Autodesk Fusion 360 part; units mm, degrees
note: some values were not read from the file. Set by a fixed rule: which sketch regions a step uses.
(part 2 of 2)
  spline S32 degree 5 poles (9.6095, -4.902) (9.5996, -4.9074) (9.5799, -4.9184) (9.5504, -4.9349) (9.5113, -4.9571) (9.4627, -4.9851) (9.4143, -5.0134) (9.3662, -5.0419) (9.3184, -5.0706) (9.2709, -5.0997) (9.2236, -5.1289) (9.1767, -5.1585) (9.1301, -5.1883) (9.0838, -5.2184) (9.0377, -5.2487) (8.992, -5.2793) (8.9466, -5.3102) (8.9016, -5.3413) (8.8568, -5.3727) (8.8124, -5.4044) (8.7683, -5.4364) (8.7246, -5.4686) (8.6812, -5.5011) (8.6382, -5.5339) (8.5955, -5.5669) (8.5532, -5.6003) (8.5113, -5.6339) (8.4697, -5.6678) (8.4286, -5.702) (8.3878, -5.7365) (8.3474, -5.7713) (8.3075, -5.8064) (8.268, -5.8419) (8.229, -5.8776) (8.1904, -5.9136) (8.1523, -5.95) (8.1146, -5.9867) (8.0774, -6.0237) (8.0407, -6.0611) (8.0046, -6.0988) (7.9691, -6.1369) (7.9341, -6.1755) (7.8999, -6.2144) (7.8664, -6.2538) (7.8337, -6.2937) (7.8017, -6.3341) (7.7767, -6.3667) (7.7583, -6.3914) (7.7462, -6.408) (7.7402, -6.4163) knots -1 -1 -1 -1 -1 -1 -0.977778 -0.955556 -0.933333 -0.911111 -0.888889 -0.866667 -0.844444 -0.822222 -0.8 -0.777778 -0.755556 -0.733333 -0.711111 -0.688889 -0.666667 -0.644444 -0.622222 -0.6 -0.577778 -0.555556 -0.533333 -0.511111 -0.488889 -0.466667 -0.444444 -0.422222 -0.4 -0.377778 -0.355556 -0.333333 -0.311111 -0.288889 -0.266667 -0.244444 -0.222222 -0.2 -0.177778 -0.155556 -0.133333 -0.111111 -0.088889 -0.066667 -0.044444 -0.022222 0 0 0 0 0 0
  arc A33 (7.7402, -6.4163) -> (6.5319, -5.8168) centre (0, -20.5) ccw
  spline S33 degree 5 poles (6.5319, -5.8168) (6.5348, -5.807) (6.5407, -5.7873) (6.5493, -5.7577) (6.5602, -5.7181) (6.5729, -5.6682) (6.5849, -5.618) (6.596, -5.5675) (6.6063, -5.5167) (6.6159, -5.4656) (6.6247, -5.4142) (6.6329, -5.3626) (6.6405, -5.3108) (6.6475, -5.2588) (6.6539, -5.2066) (6.6598, -5.1543) (6.6652, -5.1017) (6.67, -5.049) (6.6743, -4.9962) (6.6781, -4.9431) (6.6814, -4.8899) (6.6842, -4.8366) (6.6865, -4.7831) (6.6884, -4.7295) (6.6898, -4.6758) (6.6908, -4.6219) (6.6913, -4.568) (6.6914, -4.5139) (6.691, -4.4597) (6.6902, -4.4053) (6.689, -4.3509) (6.6873, -4.2964) (6.6853, -4.2418) (6.6828, -4.187) (6.6799, -4.1322) (6.6766, -4.0773) (6.6729, -4.0223) (6.6689, -3.9672) (6.6644, -3.9121) (6.6595, -3.8568) (6.6543, -3.8015) (6.6486, -3.7461) (6.6426, -3.6906) (6.6362, -3.6351) (6.6295, -3.5795) (6.6223, -3.5238) (6.6163, -3.4792) (6.6117, -3.4458) (6.6085, -3.4234) (6.6068, -3.4123) knots 0 0 0 0 0 0 0.022222 0.044444 0.066667 0.088889 0.111111 0.133333 0.155556 0.177778 0.2 0.222222 0.244444 0.266667 0.288889 0.311111 0.333333 0.355556 0.377778 0.4 0.422222 0.444444 0.466667 0.488889 0.511111 0.533333 0.555556 0.577778 0.6 0.622222 0.644444 0.666667 0.688889 0.711111 0.733333 0.755556 0.777778 0.8 0.822222 0.844444 0.866667 0.888889 0.911111 0.933333 0.955556 0.977778 1 1 1 1 1 1
  arc A34 (6.6068, -3.4123) -> (6.1565, -3.2449) centre (0, -20.5) ccw
  spline S34 degree 5 poles (6.1565, -3.2449) (6.148, -3.2523) (6.131, -3.2671) (6.1056, -3.2894) (6.0719, -3.3193) (6.0301, -3.3568) (5.9887, -3.3944) (5.9476, -3.4323) (5.9068, -3.4704) (5.8664, -3.5087) (5.8263, -3.5471) (5.7865, -3.5858) (5.7471, -3.6247) (5.708, -3.6637) (5.6693, -3.703) (5.631, -3.7424) (5.593, -3.782) (5.5554, -3.8219) (5.5181, -3.8619) (5.4813, -3.9021) (5.4448, -3.9425) (5.4087, -3.9831) (5.3731, -4.0239) (5.3378, -4.0649) (5.3029, -4.1062) (5.2685, -4.1476) (5.2344, -4.1892) (5.2009, -4.231) (5.1677, -4.273) (5.135, -4.3152) (5.1028, -4.3577) (5.071, -4.4003) (5.0397, -4.4431) (5.009, -4.4862) (4.9787, -4.5295) (4.949, -4.573) (4.9198, -4.6167) (4.8911, -4.6607) (4.863, -4.7049) (4.8355, -4.7493) (4.8087, -4.794) (4.7825, -4.8389) (4.7571, -4.8841) (4.7326, -4.9296) (4.7088, -4.9754) (4.6859, -5.0216) (4.6683, -5.0587) (4.6554, -5.0867) (4.6471, -5.1054) (4.6429, -5.1148) knots -1 -1 -1 -1 -1 -1 -0.977778 -0.955556 -0.933333 -0.911111 -0.888889 -0.866667 -0.844444 -0.822222 -0.8 -0.777778 -0.755556 -0.733333 -0.711111 -0.688889 -0.666667 -0.644444 -0.622222 -0.6 -0.577778 -0.555556 -0.533333 -0.511111 -0.488889 -0.466667 -0.444444 -0.422222 -0.4 -0.377778 -0.355556 -0.333333 -0.311111 -0.288889 -0.266667 -0.244444 -0.222222 -0.2 -0.177778 -0.155556 -0.133333 -0.111111 -0.088889 -0.066667 -0.044444 -0.022222 0 0 0 0 0 0
  arc A35 (4.6429, -5.1148) -> (3.3363, -4.7796) centre (0, -20.5) ccw
  spline S35 degree 5 poles (3.3363, -4.7796) (3.3372, -4.7694) (3.3389, -4.749) (3.3411, -4.7182) (3.3435, -4.6772) (3.3456, -4.6257) (3.3469, -4.5742) (3.3472, -4.5224) (3.3467, -4.4706) (3.3455, -4.4186) (3.3434, -4.3665) (3.3407, -4.3144) (3.3373, -4.2621) (3.3334, -4.2098) (3.3288, -4.1574) (3.3237, -4.105) (3.318, -4.0525) (3.3118, -3.9999) (3.305, -3.9473) (3.2977, -3.8946) (3.2899, -3.8419) (3.2815, -3.7892) (3.2727, -3.7364) (3.2634, -3.6836) (3.2536, -3.6307) (3.2433, -3.5778) (3.2326, -3.5249) (3.2214, -3.472) (3.2098, -3.4191) (3.1977, -3.3661) (3.1852, -3.3131) (3.1723, -3.2601) (3.1589, -3.2071) (3.1451, -3.1541) (3.1309, -3.1011) (3.1163, -3.048) (3.1012, -2.995) (3.0858, -2.942) (3.0699, -2.8889) (3.0537, -2.8359) (3.0371, -2.7829) (3.02, -2.7299) (3.0026, -2.6769) (2.9848, -2.6239) (2.9666, -2.5709) (2.9481, -2.5179) (2.9329, -2.4756) (2.9214, -2.4438) (2.9136, -2.4226) (2.9097, -2.412) knots 0 0 0 0 0 0 0.022222 0.044444 0.066667 0.088889 0.111111 0.133333 0.155556 0.177778 0.2 0.222222 0.244444 0.266667 0.288889 0.311111 0.333333 0.355556 0.377778 0.4 0.422222 0.444444 0.466667 0.488889 0.511111 0.533333 0.555556 0.577778 0.6 0.622222 0.644444 0.666667 0.688889 0.711111 0.733333 0.755556 0.777778 0.8 0.822222 0.844444 0.866667 0.888889 0.911111 0.933333 0.955556 0.977778 1 1 1 1 1 1
  arc A36 (2.9097, -2.412) -> (2.4344, -2.342) centre (0, -20.5) ccw
  spline S36 degree 5 poles (2.4344, -2.342) (2.4276, -2.351) (2.4141, -2.369) (2.3939, -2.3961) (2.3671, -2.4323) (2.3341, -2.4776) (2.3014, -2.5231) (2.2691, -2.5687) (2.2371, -2.6144) (2.2055, -2.6603) (2.1742, -2.7063) (2.1434, -2.7523) (2.1129, -2.7985) (2.0828, -2.8449) (2.0531, -2.8913) (2.0238, -2.9378) (1.9949, -2.9845) (1.9664, -3.0313) (1.9383, -3.0782) (1.9106, -3.1252) (1.8833, -3.1723) (1.8565, -3.2195) (1.8301, -3.2669) (1.8041, -3.3143) (1.7786, -3.3619) (1.7535, -3.4095) (1.7288, -3.4573) (1.7047, -3.5052) (1.681, -3.5532) (1.6578, -3.6013) (1.6351, -3.6495) (1.6129, -3.6978) (1.5912, -3.7462) (1.5701, -3.7947) (1.5495, -3.8434) (1.5294, -3.8921) (1.51, -3.9409) (1.4911, -3.9899) (1.4727, -4.039) (1.4551, -4.0881) (1.4381, -4.1374) (1.4219, -4.1868) (1.4065, -4.2363) (1.3919, -4.2859) (1.3782, -4.3357) (1.3654, -4.3855) (1.3559, -4.4255) (1.3491, -4.4556) (1.3448, -4.4756) (1.3427, -4.4857) knots -1 -1 -1 -1 -1 -1 -0.977778 -0.955556 -0.933333 -0.911111 -0.888889 -0.866667 -0.844444 -0.822222 -0.8 -0.777778 -0.755556 -0.733333 -0.711111 -0.688889 -0.666667 -0.644444 -0.622222 -0.6 -0.577778 -0.555556 -0.533333 -0.511111 -0.488889 -0.466667 -0.444444 -0.422222 -0.4 -0.377778 -0.355556 -0.333333 -0.311111 -0.288889 -0.266667 -0.244444 -0.222222 -0.2 -0.177778 -0.155556 -0.133333 -0.111111 -0.088889 -0.066667 -0.044444 -0.022222 0 0 0 0 0 0
  arc A37 (1.3427, -4.4857) -> (-0.005, -4.4295) centre (0, -20.5) ccw
  spline S37 degree 5 poles (-0.005, -4.4295) (-0.0063, -4.4193) (-0.0089, -4.399) (-0.0132, -4.3685) (-0.0193, -4.3278) (-0.0279, -4.277) (-0.0375, -4.2263) (-0.0478, -4.1757) (-0.0591, -4.125) (-0.0711, -4.0745) (-0.084, -4.024) (-0.0975, -3.9735) (-0.1116, -3.9231) (-0.1264, -3.8727) (-0.1417, -3.8224) (-0.1577, -3.7722) (-0.1741, -3.722) (-0.1911, -3.6719) (-0.2087, -3.6218) (-0.2268, -3.5719) (-0.2454, -3.5219) (-0.2646, -3.4721) (-0.2842, -3.4223) (-0.3043, -3.3725) (-0.3248, -3.3229) (-0.3459, -3.2733) (-0.3674, -3.2238) (-0.3893, -3.1743) (-0.4117, -3.125) (-0.4345, -3.0757) (-0.4577, -3.0264) (-0.4814, -2.9773) (-0.5055, -2.9282) (-0.53, -2.8792) (-0.555, -2.8303) (-0.5803, -2.7815) (-0.606, -2.7328) (-0.6322, -2.6841) (-0.6587, -2.6355) (-0.6856, -2.587) (-0.7129, -2.5386) (-0.7406, -2.4903) (-0.7686, -2.4421) (-0.7971, -2.3939) (-0.8259, -2.3459) (-0.855, -2.2979) (-0.8787, -2.2597) (-0.8965, -2.231) (-0.9085, -2.2119) (-0.9146, -2.2023) knots 0 0 0 0 0 0 0.022222 0.044444 0.066667 0.088889 0.111111 0.133333 0.155556 0.177778 0.2 0.222222 0.244444 0.266667 0.288889 0.311111 0.333333 0.355556 0.377778 0.4 0.422222 0.444444 0.466667 0.488889 0.511111 0.533333 0.555556 0.577778 0.6 0.622222 0.644444 0.666667 0.688889 0.711111 0.733333 0.755556 0.777778 0.8 0.822222 0.844444 0.866667 0.888889 0.911111 0.933333 0.955556 0.977778 1 1 1 1 1 1
  arc A38 (-0.9146, -2.2023) -> (-1.394, -2.2326) centre (0, -20.5) ccw
  spline S38 degree 5 poles (-1.394, -2.2326) (-1.3988, -2.2428) (-1.4083, -2.2633) (-1.4224, -2.294) (-1.4411, -2.3349) (-1.464, -2.3862) (-1.4865, -2.4375) (-1.5087, -2.4888) (-1.5304, -2.5402) (-1.5518, -2.5916) (-1.5728, -2.643) (-1.5934, -2.6945) (-1.6136, -2.7461) (-1.6334, -2.7976) (-1.6528, -2.8492) (-1.6718, -2.9008) (-1.6904, -2.9525) (-1.7085, -3.0042) (-1.7263, -3.0559) (-1.7436, -3.1076) (-1.7605, -3.1594) (-1.7769, -3.2112) (-1.7929, -3.263) (-1.8084, -3.3148) (-1.8235, -3.3666) (-1.8381, -3.4184) (-1.8523, -3.4703) (-1.866, -3.5221) (-1.8792, -3.574) (-1.8919, -3.6259) (-1.9041, -3.6778) (-1.9158, -3.7296) (-1.9269, -3.7815) (-1.9375, -3.8334) (-1.9475, -3.8852) (-1.957, -3.937) (-1.9659, -3.9889) (-1.9742, -4.0407) (-1.9819, -4.0925) (-1.9889, -4.1442) (-1.9953, -4.196) (-2.0009, -4.2476) (-2.0057, -4.2993) (-2.0096, -4.3508) (-2.0127, -4.4023) (-2.0148, -4.4538) (-2.0158, -4.4949) (-2.0162, -4.5257) (-2.0163, -4.5462) (-2.0162, -4.5565) knots -1 -1 -1 -1 -1 -1 -0.977778 -0.955556 -0.933333 -0.911111 -0.888889 -0.866667 -0.844444 -0.822222 -0.8 -0.777778 -0.755556 -0.733333 -0.711111 -0.688889 -0.666667 -0.644444 -0.622222 -0.6 -0.577778 -0.555556 -0.533333 -0.511111 -0.488889 -0.466667 -0.444444 -0.422222 -0.4 -0.377778 -0.355556 -0.333333 -0.311111 -0.288889 -0.266667 -0.244444 -0.222222 -0.2 -0.177778 -0.155556 -0.133333 -0.111111 -0.088889 -0.066667 -0.044444 -0.022222 0 0 0 0 0 0
  arc A39 (-2.0162, -4.5565) -> (-3.3462, -4.7817) centre (0, -20.5) ccw
  spline S39 degree 5 poles (-3.3462, -4.7817) (-3.3495, -4.772) (-3.3563, -4.7527) (-3.3668, -4.7237) (-3.3813, -4.6852) (-3.4003, -4.6374) (-3.4201, -4.5897) (-3.4408, -4.5423) (-3.4623, -4.4952) (-3.4847, -4.4482) (-3.5077, -4.4014) (-3.5314, -4.3549) (-3.5557, -4.3085) (-3.5806, -4.2624) (-3.6061, -4.2163) (-3.6321, -4.1705) (-3.6587, -4.1249) (-3.6857, -4.0794) (-3.7133, -4.0341) (-3.7414, -3.9889) (-3.77, -3.944) (-3.7991, -3.8992) (-3.8286, -3.8545) (-3.8586, -3.8101) (-3.8891, -3.7658) (-3.9199, -3.7216) (-3.9513, -3.6777) (-3.983, -3.6339) (-4.0151, -3.5902) (-4.0477, -3.5468) (-4.0807, -3.5034) (-4.1141, -3.4603) (-4.1479, -3.4173) (-4.182, -3.3745) (-4.2166, -3.3318) (-4.2515, -3.2893) (-4.2868, -3.247) (-4.3225, -3.2048) (-4.3585, -3.1628) (-4.3949, -3.121) (-4.4317, -3.0793) (-4.4688, -3.0378) (-4.5063, -2.9965) (-4.5441, -2.9553) (-4.5823, -2.9143) (-4.6208, -2.8735) (-4.6518, -2.8409) (-4.6753, -2.8166) (-4.691, -2.8004) (-4.6989, -2.7923) knots 0 0 0 0 0 0 0.022222 0.044444 0.066667 0.088889 0.111111 0.133333 0.155556 0.177778 0.2 0.222222 0.244444 0.266667 0.288889 0.311111 0.333333 0.355556 0.377778 0.4 0.422222 0.444444 0.466667 0.488889 0.511111 0.533333 0.555556 0.577778 0.6 0.622222 0.644444 0.666667 0.688889 0.711111 0.733333 0.755556 0.777778 0.8 0.822222 0.844444 0.866667 0.888889 0.911111 0.933333 0.955556 0.977778 1 1 1 1 1 1
  arc A40 (-4.6989, -2.7923) -> (-5.1616, -2.9216) centre (0, -20.5) ccw
  spline S40 degree 5 poles (-5.1616, -2.9216) (-5.1641, -2.9326) (-5.1692, -2.9546) (-5.1766, -2.9876) (-5.1863, -3.0315) (-5.1981, -3.0864) (-5.2094, -3.1412) (-5.2204, -3.1961) (-5.231, -3.2508) (-5.2413, -3.3056) (-5.2511, -3.3603) (-5.2605, -3.4149) (-5.2696, -3.4695) (-5.2782, -3.5241) (-5.2865, -3.5786) (-5.2943, -3.633) (-5.3018, -3.6874) (-5.3088, -3.7417) (-5.3154, -3.796) (-5.3216, -3.8502) (-5.3273, -3.9043) (-5.3326, -3.9584) (-5.3375, -4.0124) (-5.3419, -4.0663) (-5.3459, -4.1201) (-5.3494, -4.1739) (-5.3525, -4.2275) (-5.3551, -4.2811) (-5.3572, -4.3346) (-5.3589, -4.388) (-5.36, -4.4412) (-5.3606, -4.4944) (-5.3607, -4.5475) (-5.3603, -4.6004) (-5.3593, -4.6532) (-5.3578, -4.7059) (-5.3558, -4.7584) (-5.3531, -4.8108) (-5.3499, -4.8631) (-5.346, -4.9152) (-5.3415, -4.9671) (-5.3362, -5.0188) (-5.3302, -5.0703) (-5.3233, -5.1216) (-5.3156, -5.1726) (-5.307, -5.2234) (-5.2994, -5.2638) (-5.2934, -5.294) (-5.2892, -5.314) (-5.287, -5.3241) knots -1 -1 -1 -1 -1 -1 -0.977778 -0.955556 -0.933333 -0.911111 -0.888889 -0.866667 -0.844444 -0.822222 -0.8 -0.777778 -0.755556 -0.733333 -0.711111 -0.688889 -0.666667 -0.644444 -0.622222 -0.6 -0.577778 -0.555556 -0.533333 -0.511111 -0.488889 -0.466667 -0.444444 -0.422222 -0.4 -0.377778 -0.355556 -0.333333 -0.311111 -0.288889 -0.266667 -0.244444 -0.222222 -0.2 -0.177778 -0.155556 -0.133333 -0.111111 -0.088889 -0.066667 -0.044444 -0.022222 0 0 0 0 0 0
  arc A41 (-5.287, -5.3241) -> (-6.5411, -5.8209) centre (0, -20.5) ccw
  spline S41 degree 5 poles (-6.5411, -5.8209) (-6.5464, -5.8121) (-6.557, -5.7946) (-6.5733, -5.7685) (-6.5955, -5.7338) (-6.624, -5.691) (-6.6533, -5.6485) (-6.6834, -5.6064) (-6.7143, -5.5648) (-6.7459, -5.5235) (-6.7781, -5.4825) (-6.811, -5.4419) (-6.8444, -5.4016) (-6.8784, -5.3616) (-6.9129, -5.3219) (-6.9478, -5.2825) (-6.9833, -5.2434) (-7.0192, -5.2045) (-7.0556, -5.1659) (-7.0925, -5.1276) (-7.1298, -5.0896) (-7.1676, -5.0518) (-7.2057, -5.0143) (-7.2443, -4.977) (-7.2833, -4.94) (-7.3227, -4.9033) (-7.3625, -4.8668) (-7.4026, -4.8306) (-7.4431, -4.7946) (-7.484, -4.7588) (-7.5253, -4.7233) (-7.5669, -4.688) (-7.6089, -4.653) (-7.6512, -4.6182) (-7.6939, -4.5837) (-7.7369, -4.5494) (-7.7802, -4.5153) (-7.8239, -4.4815) (-7.8679, -4.4479) (-7.9122, -4.4145) (-7.9568, -4.3814) (-8.0018, -4.3485) (-8.047, -4.3159) (-8.0926, -4.2835) (-8.1384, -4.2513) (-8.1846, -4.2194) (-8.2217, -4.194) (-8.2497, -4.1751) (-8.2684, -4.1625) (-8.2778, -4.1562) knots 0 0 0 0 0 0 0.022222 0.044444 0.066667 0.088889 0.111111 0.133333 0.155556 0.177778 0.2 0.222222 0.244444 0.266667 0.288889 0.311111 0.333333 0.355556 0.377778 0.4 0.422222 0.444444 0.466667 0.488889 0.511111 0.533333 0.555556 0.577778 0.6 0.622222 0.644444 0.666667 0.688889 0.711111 0.733333 0.755556 0.777778 0.8 0.822222 0.844444 0.866667 0.888889 0.911111 0.933333 0.955556 0.977778 1 1 1 1 1 1
  arc A42 (-8.2778, -4.1562) -> (-8.7035, -4.3789) centre (0, -20.5) ccw
  spline S42 degree 5 poles (-8.7035, -4.3789) (-8.7037, -4.3902) (-8.7041, -4.4127) (-8.7045, -4.4465) (-8.7049, -4.4915) (-8.705, -4.5477) (-8.7047, -4.6037) (-8.704, -4.6596) (-8.703, -4.7154) (-8.7016, -4.771) (-8.6999, -4.8266) (-8.6978, -4.882) (-8.6953, -4.9373) (-8.6924, -4.9924) (-8.6891, -5.0475) (-8.6855, -5.1023) (-8.6814, -5.1571) (-8.677, -5.2117) (-8.6722, -5.2661) (-8.667, -5.3204) (-8.6613, -5.3746) (-8.6553, -5.4286) (-8.6488, -5.4824) (-8.642, -5.5361) (-8.6347, -5.5895) (-8.6269, -5.6429) (-8.6188, -5.696) (-8.6102, -5.7489) (-8.6011, -5.8017) (-8.5917, -5.8542) (-8.5817, -5.9066) (-8.5713, -5.9587) (-8.5603, -6.0106) (-8.5489, -6.0623) (-8.537, -6.1137) (-8.5245, -6.1649) (-8.5116, -6.2159) (-8.4981, -6.2666) (-8.4841, -6.3171) (-8.4695, -6.3672) (-8.4542, -6.4171) (-8.4383, -6.4666) (-8.4217, -6.5157) (-8.4043, -6.5644) (-8.3862, -6.6127) (-8.3672, -6.6606) (-8.3514, -6.6985) (-8.3392, -6.7268) (-8.3309, -6.7456) (-8.3267, -6.7549) knots -1 -1 -1 -1 -1 -1 -0.977778 -0.955556 -0.933333 -0.911111 -0.888889 -0.866667 -0.844444 -0.822222 -0.8 -0.777778 -0.755556 -0.733333 -0.711111 -0.688889 -0.666667 -0.644444 -0.622222 -0.6 -0.577778 -0.555556 -0.533333 -0.511111 -0.488889 -0.466667 -0.444444 -0.422222 -0.4 -0.377778 -0.355556 -0.333333 -0.311111 -0.288889 -0.266667 -0.244444 -0.222222 -0.2 -0.177778 -0.155556 -0.133333 -0.111111 -0.088889 -0.066667 -0.044444 -0.022222 0 0 0 0 0 0
  arc A43 (-8.3267, -6.7549) -> (-9.4501, -7.5016) centre (0, -20.5) ccw
  spline S43 degree 5 poles (-9.4501, -7.5016) (-9.4571, -7.4942) (-9.4712, -7.4792) (-9.4925, -7.457) (-9.5214, -7.4278) (-9.5582, -7.3918) (-9.5957, -7.3563) (-9.6339, -7.3214) (-9.6728, -7.2871) (-9.7122, -7.2533) (-9.7523, -7.2199) (-9.7929, -7.1871) (-9.834, -7.1546) (-9.8755, -7.1225) (-9.9175, -7.0909) (-9.9599, -7.0596) (-10.0027, -7.0287) (-10.0459, -6.9981) (-10.0896, -6.968) (-10.1336, -6.9382) (-10.178, -6.9087) (-10.2228, -6.8796) (-10.2679, -6.8509) (-10.3134, -6.8224) (-10.3593, -6.7944) (-10.4054, -6.7666) (-10.4519, -6.7392) (-10.4987, -6.7121) (-10.5458, -6.6853) (-10.5933, -6.6588) (-10.641, -6.6326) (-10.6891, -6.6068) (-10.7374, -6.5813) (-10.786, -6.5561) (-10.835, -6.5311) (-10.8842, -6.5065) (-10.9336, -6.4822) (-10.9834, -6.4582) (-11.0334, -6.4345) (-11.0837, -6.4111) (-11.1342, -6.388) (-11.185, -6.3652) (-11.236, -6.3426) (-11.2873, -6.3204) (-11.3389, -6.2985) (-11.3906, -6.2768) (-11.4323, -6.2597) (-11.4636, -6.247) (-11.4845, -6.2386) (-11.495, -6.2344) knots 0 0 0 0 0 0 0.022222 0.044444 0.066667 0.088889 0.111111 0.133333 0.155556 0.177778 0.2 0.222222 0.244444 0.266667 0.288889 0.311111 0.333333 0.355556 0.377778 0.4 0.422222 0.444444 0.466667 0.488889 0.511111 0.533333 0.555556 0.577778 0.6 0.622222 0.644444 0.666667 0.688889 0.711111 0.733333 0.755556 0.777778 0.8 0.822222 0.844444 0.866667 0.888889 0.911111 0.933333 0.955556 0.977778 1 1 1 1 1 1
  arc A44 (-11.495, -6.2344) -> (-11.8651, -6.5408) centre (0, -20.5) ccw
  spline S44 degree 5 poles (-11.8651, -6.5408) (-11.863, -6.5518) (-11.8586, -6.574) (-11.852, -6.6071) (-11.843, -6.6512) (-11.8314, -6.7061) (-11.8195, -6.7609) (-11.8072, -6.8154) (-11.7947, -6.8697) (-11.7817, -6.9239) (-11.7685, -6.9779) (-11.7549, -7.0316) (-11.7409, -7.0852) (-11.7266, -7.1386) (-11.712, -7.1917) (-11.697, -7.2446) (-11.6817, -7.2973) (-11.666, -7.3498) (-11.65, -7.4021) (-11.6336, -7.4541) (-11.6168, -7.5059) (-11.5997, -7.5575) (-11.5822, -7.6088) (-11.5643, -7.6598) (-11.546, -7.7106) (-11.5274, -7.7612) (-11.5084, -7.8114) (-11.489, -7.8614) (-11.4691, -7.9111) (-11.4489, -7.9606) (-11.4283, -8.0097) (-11.4073, -8.0585) (-11.3858, -8.107) (-11.3639, -8.1552) (-11.3415, -8.2031) (-11.3187, -8.2506) (-11.2954, -8.2977) (-11.2717, -8.3445) (-11.2475, -8.3909) (-11.2228, -8.437) (-11.1975, -8.4826) (-11.1717, -8.5277) (-11.1452, -8.5722) (-11.1181, -8.6163) (-11.0903, -8.6597) (-11.0618, -8.7026) (-11.0384, -8.7365) (-11.0206, -8.7616) (-11.0086, -8.7782) (-11.0025, -8.7865) knots -1 -1 -1 -1 -1 -1 -0.977778 -0.955556 -0.933333 -0.911111 -0.888889 -0.866667 -0.844444 -0.822222 -0.8 -0.777778 -0.755556 -0.733333 -0.711111 -0.688889 -0.666667 -0.644444 -0.622222 -0.6 -0.577778 -0.555556 -0.533333 -0.511111 -0.488889 -0.466667 -0.444444 -0.422222 -0.4 -0.377778 -0.355556 -0.333333 -0.311111 -0.288889 -0.266667 -0.244444 -0.222222 -0.2 -0.177778 -0.155556 -0.133333 -0.111111 -0.088889 -0.066667 -0.044444 -0.022222 0 0 0 0 0 0
  arc A45 (-11.0025, -8.7865) -> (-11.9461, -9.7505) centre (0, -20.5) ccw
  spline S45 degree 5 poles (-11.9461, -9.7505) (-11.9545, -9.7446) (-11.9714, -9.7329) (-11.9969, -9.7157) (-12.0312, -9.6931) (-12.0747, -9.6655) (-12.1188, -9.6386) (-12.1634, -9.6124) (-12.2085, -9.5869) (-12.2542, -9.562) (-12.3003, -9.5378) (-12.3468, -9.514) (-12.3937, -9.4908) (-12.441, -9.4681) (-12.4887, -9.4459) (-12.5367, -9.4241) (-12.585, -9.4027) (-12.6336, -9.3819) (-12.6826, -9.3614) (-12.7318, -9.3414) (-12.7814, -9.3218) (-12.8312, -9.3027) (-12.8814, -9.2839) (-12.9318, -9.2656) (-12.9824, -9.2477) (-13.0334, -9.2301) (-13.0845, -9.2129) (-13.136, -9.1962) (-13.1876, -9.1798) (-13.2395, -9.1637) (-13.2917, -9.1481) (-13.344, -9.1328) (-13.3966, -9.1179) (-13.4495, -9.1033) (-13.5025, -9.0891) (-13.5557, -9.0753) (-13.6092, -9.0618) (-13.6628, -9.0486) (-13.7167, -9.0358) (-13.7707, -9.0234) (-13.8249, -9.0113) (-13.8794, -8.9995) (-13.934, -8.9881) (-13.9888, -8.977) (-14.0437, -8.9663) (-14.0989, -8.9559) (-14.1432, -8.9478) (-14.1764, -8.9419) (-14.1987, -8.938) (-14.2098, -8.9361) knots 0 0 0 0 0 0 0.022222 0.044444 0.066667 0.088889 0.111111 0.133333 0.155556 0.177778 0.2 0.222222 0.244444 0.266667 0.288889 0.311111 0.333333 0.355556 0.377778 0.4 0.422222 0.444444 0.466667 0.488889 0.511111 0.533333 0.555556 0.577778 0.6 0.622222 0.644444 0.666667 0.688889 0.711111 0.733333 0.755556 0.777778 0.8 0.822222 0.844444 0.866667 0.888889 0.911111 0.933333 0.955556 0.977778 1 1 1 1 1 1
  arc A46 (-14.2098, -8.9361) -> (-14.5081, -9.3127) centre (0, -20.5) ccw
  spline S46 degree 5 poles (-14.5081, -9.3127) (-14.5037, -9.3231) (-14.4949, -9.3438) (-14.4815, -9.3749) (-14.4635, -9.4161) (-14.4408, -9.4674) (-14.4177, -9.5185) (-14.3944, -9.5693) (-14.3708, -9.6199) (-14.3469, -9.6701) (-14.3227, -9.7202) (-14.2982, -9.7699) (-14.2735, -9.8194) (-14.2484, -9.8686) (-14.223, -9.9176) (-14.1974, -9.9662) (-14.1714, -10.0146) (-14.1452, -10.0627) (-14.1186, -10.1105) (-14.0917, -10.158) (-14.0646, -10.2051) (-14.0371, -10.252) (-14.0093, -10.2985) (-13.9812, -10.3448) (-13.9528, -10.3907) (-13.924, -10.4362) (-13.895, -10.4814) (-13.8656, -10.5263) (-13.8359, -10.5708) (-13.8058, -10.615) (-13.7754, -10.6587) (-13.7447, -10.7021) (-13.7136, -10.7451) (-13.6821, -10.7877) (-13.6503, -10.8298) (-13.6181, -10.8715) (-13.5856, -10.9128) (-13.5526, -10.9537) (-13.5193, -10.994) (-13.4856, -11.0339) (-13.4514, -11.0733) (-13.4167, -11.112) (-13.3816, -11.1501) (-13.3459, -11.1875) (-13.3096, -11.2243) (-13.2728, -11.2603) (-13.243, -11.2886) (-13.2203, -11.3094) (-13.2051, -11.3232) (-13.1975, -11.3301) knots -1 -1 -1 -1 -1 -1 -0.977778 -0.955556 -0.933333 -0.911111 -0.888889 -0.866667 -0.844444 -0.822222 -0.8 -0.777778 -0.755556 -0.733333 -0.711111 -0.688889 -0.666667 -0.644444 -0.622222 -0.6 -0.577778 -0.555556 -0.533333 -0.511111 -0.488889 -0.466667 -0.444444 -0.422222 -0.4 -0.377778 -0.355556 -0.333333 -0.311111 -0.288889 -0.266667 -0.244444 -0.222222 -0.2 -0.177778 -0.155556 -0.133333 -0.111111 -0.088889 -0.066667 -0.044444 -0.022222 0 0 0 0 0 0
  arc A47 (-13.1975, -11.3301) -> (-13.92, -12.4691) centre (0, -20.5) ccw
  spline S47 degree 5 poles (-13.92, -12.4691) (-13.9294, -12.4651) (-13.9484, -12.4572) (-13.9769, -12.4456) (-14.0152, -12.4306) (-14.0635, -12.4127) (-14.1121, -12.3956) (-14.1612, -12.3793) (-14.2107, -12.3637) (-14.2605, -12.3488) (-14.3107, -12.3347) (-14.3611, -12.3212) (-14.4118, -12.3082) (-14.4628, -12.2958) (-14.5141, -12.284) (-14.5655, -12.2726) (-14.6172, -12.2618) (-14.6691, -12.2515) (-14.7213, -12.2417) (-14.7736, -12.2323) (-14.8262, -12.2235) (-14.8789, -12.2151) (-14.9318, -12.2072) (-14.9849, -12.1998) (-15.0382, -12.1928) (-15.0917, -12.1862) (-15.1453, -12.18) (-15.1991, -12.1743) (-15.2531, -12.169) (-15.3072, -12.1641) (-15.3614, -12.1596) (-15.4158, -12.1556) (-15.4704, -12.1519) (-15.5251, -12.1487) (-15.5799, -12.1458) (-15.6348, -12.1433) (-15.6899, -12.1412) (-15.7451, -12.1395) (-15.8004, -12.1382) (-15.8559, -12.1373) (-15.9115, -12.1367) (-15.9671, -12.1365) (-16.0229, -12.1367) (-16.0788, -12.1372) (-16.1348, -12.1382) (-16.191, -12.1394) (-16.2359, -12.1408) (-16.2697, -12.1419) (-16.2922, -12.1428) (-16.3035, -12.1432) knots 0 0 0 0 0 0 0.022222 0.044444 0.066667 0.088889 0.111111 0.133333 0.155556 0.177778 0.2 0.222222 0.244444 0.266667 0.288889 0.311111 0.333333 0.355556 0.377778 0.4 0.422222 0.444444 0.466667 0.488889 0.511111 0.533333 0.555556 0.577778 0.6 0.622222 0.644444 0.666667 0.688889 0.711111 0.733333 0.755556 0.777778 0.8 0.822222 0.844444 0.866667 0.888889 0.911111 0.933333 0.955556 0.977778 1 1 1 1 1 1
  arc A48 (-16.3035, -12.1432) -> (-16.5171, -12.5736) centre (0, -20.5) ccw
  spline S48 degree 5 poles (-16.5171, -12.5736) (-16.5106, -12.5828) (-16.4976, -12.6013) (-16.4781, -12.6289) (-16.4519, -12.6655) (-16.419, -12.7109) (-16.3859, -12.7561) (-16.3525, -12.8009) (-16.3189, -12.8455) (-16.285, -12.8897) (-16.251, -12.9336) (-16.2167, -12.9772) (-16.1822, -13.0204) (-16.1474, -13.0634) (-16.1124, -13.106) (-16.0772, -13.1482) (-16.0418, -13.1901) (-16.0061, -13.2317) (-15.9702, -13.2729) (-15.934, -13.3138) (-15.8976, -13.3543) (-15.861, -13.3944) (-15.8242, -13.4342) (-15.7871, -13.4735) (-15.7497, -13.5125) (-15.7121, -13.5511) (-15.6743, -13.5893) (-15.6362, -13.6271) (-15.5979, -13.6644) (-15.5594, -13.7014) (-15.5205, -13.7379) (-15.4814, -13.7739) (-15.4421, -13.8095) (-15.4025, -13.8446) (-15.3626, -13.8792) (-15.3224, -13.9133) (-15.282, -13.9469) (-15.2413, -13.98) (-15.2003, -14.0126) (-15.159, -14.0446) (-15.1174, -14.076) (-15.0754, -14.1066) (-15.0331, -14.1366) (-14.9904, -14.1658) (-14.9473, -14.1942) (-14.9038, -14.2218) (-14.8687, -14.2432) (-14.8422, -14.2589) (-14.8245, -14.2692) (-14.8156, -14.2743) knots -1 -1 -1 -1 -1 -1 -0.977778 -0.955556 -0.933333 -0.911111 -0.888889 -0.866667 -0.844444 -0.822222 -0.8 -0.777778 -0.755556 -0.733333 -0.711111 -0.688889 -0.666667 -0.644444 -0.622222 -0.6 -0.577778 -0.555556 -0.533333 -0.511111 -0.488889 -0.466667 -0.444444 -0.422222 -0.4 -0.377778 -0.355556 -0.333333 -0.311111 -0.288889 -0.266667 -0.244444 -0.222222 -0.2 -0.177778 -0.155556 -0.133333 -0.111111 -0.088889 -0.066667 -0.044444 -0.022222 0 0 0 0 0 0
  arc A49 (-14.8156, -14.2743) -> (-15.2855, -15.5387) centre (0, -20.5) ccw
  spline S49 degree 5 poles (-15.2855, -15.5387) (-15.2956, -15.5368) (-15.3158, -15.533) (-15.3461, -15.5276) (-15.3866, -15.5209) (-15.4376, -15.5134) (-15.4888, -15.5068) (-15.5402, -15.501) (-15.5918, -15.4961) (-15.6436, -15.4919) (-15.6956, -15.4885) (-15.7478, -15.4857) (-15.8001, -15.4836) (-15.8525, -15.4821) (-15.9051, -15.4812) (-15.9578, -15.4808) (-16.0106, -15.4809) (-16.0635, -15.4816) (-16.1166, -15.4829) (-16.1697, -15.4846) (-16.2229, -15.4869) (-16.2763, -15.4897) (-16.3297, -15.493) (-16.3832, -15.4967) (-16.4368, -15.5009) (-16.4904, -15.5056) (-16.5442, -15.5107) (-16.598, -15.5163) (-16.6519, -15.5223) (-16.7058, -15.5288) (-16.7598, -15.5357) (-16.8139, -15.5431) (-16.868, -15.5508) (-16.9221, -15.559) (-16.9764, -15.5676) (-17.0306, -15.5766) (-17.0849, -15.586) (-17.1393, -15.5958) (-17.1937, -15.606) (-17.2481, -15.6166) (-17.3026, -15.6276) (-17.3571, -15.639) (-17.4116, -15.6508) (-17.4662, -15.663) (-17.5208, -15.6755) (-17.5754, -15.6884) (-17.6191, -15.6991) (-17.6519, -15.7072) (-17.6738, -15.7127) (-17.6847, -15.7155) knots 0 0 0 0 0 0 0.022222 0.044444 0.066667 0.088889 0.111111 0.133333 0.155556 0.177778 0.2 0.222222 0.244444 0.266667 0.288889 0.311111 0.333333 0.355556 0.377778 0.4 0.422222 0.444444 0.466667 0.488889 0.511111 0.533333 0.555556 0.577778 0.6 0.622222 0.644444 0.666667 0.688889 0.711111 0.733333 0.755556 0.777778 0.8 0.822222 0.844444 0.866667 0.888889 0.911111 0.933333 0.955556 0.977778 1 1 1 1 1 1
  arc A50 (-17.6847, -15.7155) -> (-17.8041, -16.1809) centre (0, -20.5) ccw
  spline S50 degree 5 poles (-17.8041, -16.1809) (-17.7959, -16.1886) (-17.7793, -16.2039) (-17.7545, -16.2269) (-17.7213, -16.2572) (-17.6797, -16.2948) (-17.6378, -16.3321) (-17.5959, -16.369) (-17.5537, -16.4056) (-17.5114, -16.4418) (-17.469, -16.4777) (-17.4264, -16.5132) (-17.3836, -16.5484) (-17.3407, -16.5831) (-17.2976, -16.6175) (-17.2544, -16.6515) (-17.211, -16.6852) (-17.1675, -16.7184) (-17.1238, -16.7512) (-17.0799, -16.7837) (-17.0359, -16.8157) (-16.9918, -16.8474) (-16.9474, -16.8786) (-16.903, -16.9094) (-16.8583, -16.9398) (-16.8136, -16.9697) (-16.7686, -16.9992) (-16.7235, -17.0282) (-16.6783, -17.0568) (-16.6329, -17.0849) (-16.5873, -17.1125) (-16.5416, -17.1397) (-16.4957, -17.1663) (-16.4496, -17.1924) (-16.4034, -17.2179) (-16.357, -17.2429) (-16.3105, -17.2674) (-16.2638, -17.2913) (-16.2169, -17.3147) (-16.1699, -17.3374) (-16.1227, -17.3594) (-16.0752, -17.3807) (-16.0276, -17.4012) (-15.9798, -17.4209) (-15.9317, -17.4397) (-15.8835, -17.4577) (-15.8447, -17.4713) (-15.8155, -17.4812) (-15.796, -17.4876) (-15.7862, -17.4907) knots -1 -1 -1 -1 -1 -1 -0.977778 -0.955556 -0.933333 -0.911111 -0.888889 -0.866667 -0.844444 -0.822222 -0.8 -0.777778 -0.755556 -0.733333 -0.711111 -0.688889 -0.666667 -0.644444 -0.622222 -0.6 -0.577778 -0.555556 -0.533333 -0.511111 -0.488889 -0.466667 -0.444444 -0.422222 -0.4 -0.377778 -0.355556 -0.333333 -0.311111 -0.288889 -0.266667 -0.244444 -0.222222 -0.2 -0.177778 -0.155556 -0.133333 -0.111111 -0.088889 -0.066667 -0.044444 -0.022222 0 0 0 0 0 0
  arc A51 (-15.7862, -17.4907) -> (-15.983, -18.8252) centre (0, -20.5) ccw
  spline S51 degree 5 poles (-15.983, -18.8252) (-15.9933, -18.8254) (-16.0138, -18.8259) (-16.0445, -18.8269) (-16.0856, -18.8288) (-16.137, -18.832) (-16.1884, -18.8362) (-16.2399, -18.8412) (-16.2914, -18.8471) (-16.343, -18.8538) (-16.3946, -18.8613) (-16.4462, -18.8694) (-16.4978, -18.8783) (-16.5494, -18.8877) (-16.601, -18.8977) (-16.6526, -18.9083) (-16.7043, -18.9194) (-16.7559, -18.9311) (-16.8075, -18.9433) (-16.8591, -18.9561) (-16.9107, -18.9694) (-16.9623, -18.9832) (-17.0139, -18.9975) (-17.0654, -19.0123) (-17.117, -19.0276) (-17.1685, -19.0433) (-17.22, -19.0595) (-17.2714, -19.0761) (-17.3229, -19.0932) (-17.3743, -19.1108) (-17.4257, -19.1288) (-17.477, -19.1472) (-17.5284, -19.166) (-17.5796, -19.1853) (-17.6309, -19.205) (-17.6821, -19.225) (-17.7333, -19.2455) (-17.7844, -19.2664) (-17.8355, -19.2877) (-17.8865, -19.3094) (-17.9375, -19.3315) (-17.9885, -19.354) (-18.0393, -19.3769) (-18.0902, -19.4001) (-18.141, -19.4237) (-18.1917, -19.4477) (-18.2323, -19.4672) (-18.2627, -19.482) (-18.2829, -19.4919) (-18.293, -19.4969) knots 0 0 0 0 0 0 0.022222 0.044444 0.066667 0.088889 0.111111 0.133333 0.155556 0.177778 0.2 0.222222 0.244444 0.266667 0.288889 0.311111 0.333333 0.355556 0.377778 0.4 0.422222 0.444444 0.466667 0.488889 0.511111 0.533333 0.555556 0.577778 0.6 0.622222 0.644444 0.666667 0.688889 0.711111 0.733333 0.755556 0.777778 0.8 0.822222 0.844444 0.866667 0.888889 0.911111 0.933333 0.955556 0.977778 1 1 1 1 1 1
  arc A52 (-18.293, -19.4969) -> (-18.313, -19.9769) centre (0, -20.5) ccw
  spline S52 degree 5 poles (-18.313, -19.9769) (-18.3034, -19.9828) (-18.284, -19.9943) (-18.255, -20.0116) (-18.2162, -20.0344) (-18.1676, -20.0625) (-18.119, -20.0903) (-18.0702, -20.1177) (-18.0214, -20.1447) (-17.9725, -20.1714) (-17.9235, -20.1976) (-17.8745, -20.2235) (-17.8254, -20.249) (-17.7761, -20.274) (-17.7269, -20.2987) (-17.6775, -20.323) (-17.6281, -20.3469) (-17.5786, -20.3704) (-17.529, -20.3934) (-17.4794, -20.416) (-17.4296, -20.4382) (-17.3799, -20.46) (-17.33, -20.4813) (-17.2801, -20.5022) (-17.2302, -20.5226) (-17.1801, -20.5426) (-17.13, -20.5621) (-17.0799, -20.5811) (-17.0297, -20.5996) (-16.9794, -20.6177) (-16.9291, -20.6353) (-16.8788, -20.6523) (-16.8283, -20.6688) (-16.7779, -20.6847) (-16.7273, -20.7001) (-16.6768, -20.7149) (-16.6262, -20.7292) (-16.5755, -20.7429) (-16.5248, -20.756) (-16.4741, -20.7684) (-16.4233, -20.7801) (-16.3725, -20.7911) (-16.3216, -20.8013) (-16.2708, -20.8106) (-16.2198, -20.819) (-16.1689, -20.8265) (-16.1281, -20.8318) (-16.0975, -20.8354) (-16.0771, -20.8376) (-16.0669, -20.8386) knots -1 -1 -1 -1 -1 -1 -0.977778 -0.955556 -0.933333 -0.911111 -0.888889 -0.866667 -0.844444 -0.822222 -0.8 -0.777778 -0.755556 -0.733333 -0.711111 -0.688889 -0.666667 -0.644444 -0.622222 -0.6 -0.577778 -0.555556 -0.533333 -0.511111 -0.488889 -0.466667 -0.444444 -0.422222 -0.4 -0.377778 -0.355556 -0.333333 -0.311111 -0.288889 -0.266667 -0.244444 -0.222222 -0.2 -0.177778 -0.155556 -0.133333 -0.111111 -0.088889 -0.066667 -0.044444 -0.022222 0 0 0 0 0 0
  arc A53 (-16.0669, -20.8386) -> (-15.9819, -22.1848) centre (0, -20.5) ccw
  spline S53 degree 5 poles (-15.9819, -22.1848) (-15.9919, -22.1872) (-16.0119, -22.1919) (-16.0418, -22.1993) (-16.0816, -22.2097) (-16.1312, -22.2236) (-16.1806, -22.2383) (-16.2299, -22.2539) (-16.2791, -22.2704) (-16.3281, -22.2877) (-16.377, -22.3057) (-16.4258, -22.3244) (-16.4744, -22.3438) (-16.523, -22.3637) (-16.5714, -22.3842) (-16.6197, -22.4053) (-16.6679, -22.4269) (-16.7159, -22.4491) (-16.7639, -22.4718) (-16.8117, -22.495) (-16.8594, -22.5188) (-16.907, -22.543) (-16.9545, -22.5677) (-17.0018, -22.5929) (-17.0491, -22.6186) (-17.0962, -22.6447) (-17.1432, -22.6712) (-17.1901, -22.6982) (-17.2368, -22.7256) (-17.2835, -22.7535) (-17.33, -22.7817) (-17.3764, -22.8104) (-17.4227, -22.8395) (-17.4688, -22.869) (-17.5149, -22.8989) (-17.5608, -22.9292) (-17.6066, -22.9599) (-17.6522, -22.991) (-17.6978, -23.0224) (-17.7432, -23.0543) (-17.7885, -23.0865) (-17.8336, -23.119) (-17.8787, -23.152) (-17.9236, -23.1853) (-17.9683, -23.219) (-18.013, -23.253) (-18.0486, -23.2805) (-18.0752, -23.3013) (-18.093, -23.3152) (-18.1018, -23.3222) knots 0 0 0 0 0 0 0.022222 0.044444 0.066667 0.088889 0.111111 0.133333 0.155556 0.177778 0.2 0.222222 0.244444 0.266667 0.288889 0.311111 0.333333 0.355556 0.377778 0.4 0.422222 0.444444 0.466667 0.488889 0.511111 0.533333 0.555556 0.577778 0.6 0.622222 0.644444 0.666667 0.688889 0.711111 0.733333 0.755556 0.777778 0.8 0.822222 0.844444 0.866667 0.888889 0.911111 0.933333 0.955556 0.977778 1 1 1 1 1 1
  arc A54 (-18.1018, -23.3222) -> (-18.0216, -23.7959) centre (0, -20.5) ccw
  spline S54 degree 5 poles (-18.0216, -23.7959) (-18.0109, -23.7995) (-17.9896, -23.8069) (-17.9576, -23.8177) (-17.9149, -23.8319) (-17.8616, -23.8494) (-17.8082, -23.8664) (-17.7548, -23.8831) (-17.7015, -23.8993) (-17.6481, -23.9152) (-17.5947, -23.9307) (-17.5414, -23.9458) (-17.488, -23.9605) (-17.4347, -23.9749) (-17.3813, -23.9888) (-17.328, -24.0022) (-17.2747, -24.0153) (-17.2214, -24.028) (-17.1681, -24.0402) (-17.1148, -24.052) (-17.0616, -24.0634) (-17.0084, -24.0743) (-16.9552, -24.0848) (-16.9021, -24.0949) (-16.8489, -24.1045) (-16.7959, -24.1136) (-16.7428, -24.1222) (-16.6898, -24.1304) (-16.6368, -24.1381) (-16.5839, -24.1454) (-16.5311, -24.1521) (-16.4783, -24.1582) (-16.4255, -24.1639) (-16.3728, -24.169) (-16.3202, -24.1735) (-16.2677, -24.1775) (-16.2152, -24.181) (-16.1628, -24.1838) (-16.1105, -24.1861) (-16.0583, -24.1877) (-16.0062, -24.1886) (-15.9542, -24.1888) (-15.9023, -24.1881) (-15.8506, -24.1867) (-15.7991, -24.1843) (-15.7477, -24.1811) (-15.7067, -24.1778) (-15.676, -24.1749) (-15.6556, -24.1728) (-15.6454, -24.1717) knots -1 -1 -1 -1 -1 -1 -0.977778 -0.955556 -0.933333 -0.911111 -0.888889 -0.866667 -0.844444 -0.822222 -0.8 -0.777778 -0.755556 -0.733333 -0.711111 -0.688889 -0.666667 -0.644444 -0.622222 -0.6 -0.577778 -0.555556 -0.533333 -0.511111 -0.488889 -0.466667 -0.444444 -0.422222 -0.4 -0.377778 -0.355556 -0.333333 -0.311111 -0.288889 -0.266667 -0.244444 -0.222222 -0.2 -0.177778 -0.155556 -0.133333 -0.111111 -0.088889 -0.066667 -0.044444 -0.022222 0 0 0 0 0 0
  arc A55 (-15.6454, -24.1717) -> (-15.2824, -25.4708) centre (0, -20.5) ccw
  spline S55 degree 5 poles (-15.2824, -25.4708) (-15.2917, -25.4752) (-15.3102, -25.484) (-15.3379, -25.4974) (-15.3747, -25.5159) (-15.4203, -25.5397) (-15.4656, -25.5645) (-15.5106, -25.59) (-15.5553, -25.6163) (-15.5996, -25.6434) (-15.6437, -25.6712) (-15.6875, -25.6997) (-15.7311, -25.7287) (-15.7744, -25.7583) (-15.8175, -25.7885) (-15.8604, -25.8191) (-15.903, -25.8503) (-15.9454, -25.882) (-15.9876, -25.9141) (-16.0295, -25.9468) (-16.0713, -25.9799) (-16.1128, -26.0135) (-16.1541, -26.0476) (-16.1952, -26.0821) (-16.236, -26.117) (-16.2767, -26.1523) (-16.3171, -26.188) (-16.3574, -26.2242) (-16.3974, -26.2607) (-16.4373, -26.2976) (-16.4769, -26.335) (-16.5163, -26.3727) (-16.5555, -26.4108) (-16.5945, -26.4492) (-16.6334, -26.488) (-16.672, -26.5272) (-16.7104, -26.5668) (-16.7486, -26.6066) (-16.7866, -26.6469) (-16.8244, -26.6875) (-16.862, -26.7284) (-16.8994, -26.7696) (-16.9366, -26.8112) (-16.9736, -26.8531) (-17.0104, -26.8954) (-17.047, -26.9379) (-17.0761, -26.9722) (-17.0978, -26.9981) (-17.1123, -27.0154) (-17.1195, -27.0241) knots 0 0 0 0 0 0 0.022222 0.044444 0.066667 0.088889 0.111111 0.133333 0.155556 0.177778 0.2 0.222222 0.244444 0.266667 0.288889 0.311111 0.333333 0.355556 0.377778 0.4 0.422222 0.444444 0.466667 0.488889 0.511111 0.533333 0.555556 0.577778 0.6 0.622222 0.644444 0.666667 0.688889 0.711111 0.733333 0.755556 0.777778 0.8 0.822222 0.844444 0.866667 0.888889 0.911111 0.933333 0.955556 0.977778 1 1 1 1 1 1
  arc A56 (-17.1195, -27.0241) -> (-16.9425, -27.4708) centre (0, -20.5) ccw
  spline S56 degree 5 poles (-16.9425, -27.4708) (-16.9313, -27.4721) (-16.9089, -27.4748) (-16.8754, -27.4788) (-16.8307, -27.4839) (-16.7749, -27.4898) (-16.7191, -27.4954) (-16.6635, -27.5006) (-16.6079, -27.5054) (-16.5524, -27.5099) (-16.497, -27.5139) (-16.4416, -27.5176) (-16.3864, -27.5209) (-16.3312, -27.5238) (-16.2762, -27.5263) (-16.2212, -27.5284) (-16.1663, -27.5301) (-16.1116, -27.5314) (-16.0569, -27.5323) (-16.0023, -27.5328) (-15.9479, -27.5328) (-15.8936, -27.5325) (-15.8394, -27.5317) (-15.7853, -27.5305) (-15.7313, -27.5288) (-15.6775, -27.5267) (-15.6238, -27.5241) (-15.5703, -27.5211) (-15.5169, -27.5176) (-15.4636, -27.5137) (-15.4105, -27.5093) (-15.3576, -27.5043) (-15.3048, -27.4989) (-15.2522, -27.4929) (-15.1998, -27.4864) (-15.1476, -27.4794) (-15.0955, -27.4719) (-15.0437, -27.4638) (-14.9921, -27.4551) (-14.9407, -27.4458) (-14.8895, -27.4359) (-14.8386, -27.4252) (-14.788, -27.4138) (-14.7378, -27.4016) (-14.6878, -27.3886) (-14.6382, -27.3748) (-14.5988, -27.363) (-14.5694, -27.3538) (-14.5499, -27.3476) (-14.5401, -27.3444) knots -1 -1 -1 -1 -1 -1 -0.977778 -0.955556 -0.933333 -0.911111 -0.888889 -0.866667 -0.844444 -0.822222 -0.8 -0.777778 -0.755556 -0.733333 -0.711111 -0.688889 -0.666667 -0.644444 -0.622222 -0.6 -0.577778 -0.555556 -0.533333 -0.511111 -0.488889 -0.466667 -0.444444 -0.422222 -0.4 -0.377778 -0.355556 -0.333333 -0.311111 -0.288889 -0.266667 -0.244444 -0.222222 -0.2 -0.177778 -0.155556 -0.133333 -0.111111 -0.088889 -0.066667 -0.044444 -0.022222 0 0 0 0 0 0
  arc A57 (-14.5401, -27.3444) -> (-13.915, -28.5396) centre (0, -20.5) ccw
  spline S57 degree 5 poles (-13.915, -28.5396) (-13.9231, -28.5458) (-13.9394, -28.5583) (-13.9637, -28.5772) (-13.9959, -28.6028) (-14.0355, -28.6357) (-14.0747, -28.6693) (-14.1134, -28.7036) (-14.1516, -28.7387) (-14.1894, -28.7744) (-14.2267, -28.8107) (-14.2636, -28.8477) (-14.3002, -28.8851) (-14.3364, -28.9231) (-14.3723, -28.9615) (-14.4079, -29.0004) (-14.4431, -29.0398) (-14.478, -29.0796) (-14.5126, -29.1198) (-14.5468, -29.1605) (-14.5807, -29.2016) (-14.6143, -29.2431) (-14.6477, -29.285) (-14.6807, -29.3272) (-14.7134, -29.3699) (-14.7458, -29.4129) (-14.778, -29.4562) (-14.8098, -29.5) (-14.8414, -29.544) (-14.8727, -29.5884) (-14.9037, -29.6332) (-14.9344, -29.6783) (-14.9648, -29.7237) (-14.995, -29.7694) (-15.0249, -29.8155) (-15.0545, -29.8618) (-15.0839, -29.9085) (-15.1129, -29.9554) (-15.1418, -30.0027) (-15.1703, -30.0502) (-15.1986, -30.0981) (-15.2266, -30.1462) (-15.2543, -30.1946) (-15.2818, -30.2433) (-15.309, -30.2923) (-15.3359, -30.3415) (-15.3573, -30.3811) (-15.3732, -30.4109) (-15.3837, -30.4309) (-15.389, -30.4409) knots 0 0 0 0 0 0 0.022222 0.044444 0.066667 0.088889 0.111111 0.133333 0.155556 0.177778 0.2 0.222222 0.244444 0.266667 0.288889 0.311111 0.333333 0.355556 0.377778 0.4 0.422222 0.444444 0.466667 0.488889 0.511111 0.533333 0.555556 0.577778 0.6 0.622222 0.644444 0.666667 0.688889 0.711111 0.733333 0.755556 0.777778 0.8 0.822222 0.844444 0.866667 0.888889 0.911111 0.933333 0.955556 0.977778 1 1 1 1 1 1
  arc A58 (-15.389, -30.4409) -> (-15.123, -30.841) centre (0, -20.5) ccw
  spline S58 degree 5 poles (-15.123, -30.841) (-15.1118, -30.84) (-15.0893, -30.838) (-15.0556, -30.8349) (-15.0109, -30.8305) (-14.955, -30.8247) (-14.8994, -30.8186) (-14.8438, -30.8121) (-14.7885, -30.8053) (-14.7332, -30.7981) (-14.6782, -30.7906) (-14.6233, -30.7827) (-14.5686, -30.7744) (-14.514, -30.7658) (-14.4596, -30.7568) (-14.4054, -30.7474) (-14.3514, -30.7376) (-14.2976, -30.7275) (-14.2439, -30.717) (-14.1905, -30.7062) (-14.1372, -30.6949) (-14.0841, -30.6833) (-14.0313, -30.6712) (-13.9786, -30.6588) (-13.9262, -30.6459) (-13.874, -30.6327) (-13.822, -30.619) (-13.7703, -30.6049) (-13.7187, -30.5904) (-13.6675, -30.5755) (-13.6164, -30.5601) (-13.5657, -30.5443) (-13.5152, -30.528) (-13.465, -30.5112) (-13.4151, -30.494) (-13.3655, -30.4763) (-13.3161, -30.458) (-13.2671, -30.4393) (-13.2184, -30.4201) (-13.17, -30.4004) (-13.1221, -30.38) (-13.0745, -30.359) (-13.0274, -30.3373) (-12.9808, -30.315) (-12.9346, -30.2919) (-12.889, -30.268) (-12.8529, -30.2483) (-12.8261, -30.2332) (-12.8083, -30.223) (-12.7994, -30.2179) knots -1 -1 -1 -1 -1 -1 -0.977778 -0.955556 -0.933333 -0.911111 -0.888889 -0.866667 -0.844444 -0.822222 -0.8 -0.777778 -0.755556 -0.733333 -0.711111 -0.688889 -0.666667 -0.644444 -0.622222 -0.6 -0.577778 -0.555556 -0.533333 -0.511111 -0.488889 -0.466667 -0.444444 -0.422222 -0.4 -0.377778 -0.355556 -0.333333 -0.311111 -0.288889 -0.266667 -0.244444 -0.222222 -0.2 -0.177778 -0.155556 -0.133333 -0.111111 -0.088889 -0.066667 -0.044444 -0.022222 0 0 0 0 0 0
  arc A59 (-12.7994, -30.2179) -> (-11.9393, -31.257) centre (0, -20.5) ccw
  spline S59 degree 5 poles (-11.9393, -31.257) (-11.9461, -31.2648) (-11.9594, -31.2803) (-11.9793, -31.3039) (-12.0053, -31.3357) (-12.0373, -31.376) (-12.0686, -31.417) (-12.0993, -31.4587) (-12.1294, -31.5009) (-12.1589, -31.5437) (-12.1879, -31.587) (-12.2164, -31.6308) (-12.2444, -31.6751) (-12.2719, -31.7197) (-12.299, -31.7648) (-12.3257, -31.8102) (-12.352, -31.8561) (-12.3778, -31.9022) (-12.4033, -31.9488) (-12.4283, -31.9957) (-12.4529, -32.0429) (-12.4772, -32.0905) (-12.5011, -32.1384) (-12.5246, -32.1866) (-12.5477, -32.2351) (-12.5705, -32.2839) (-12.5929, -32.333) (-12.615, -32.3824) (-12.6367, -32.4321) (-12.6581, -32.482) (-12.6791, -32.5323) (-12.6998, -32.5828) (-12.7201, -32.6335) (-12.7401, -32.6845) (-12.7598, -32.7357) (-12.7791, -32.7872) (-12.7981, -32.839) (-12.8168, -32.891) (-12.8351, -32.9432) (-12.8532, -32.9956) (-12.8709, -33.0483) (-12.8883, -33.1012) (-12.9053, -33.1543) (-12.9221, -33.2077) (-12.9385, -33.2612) (-12.9546, -33.315) (-12.9673, -33.3581) (-12.9766, -33.3906) (-12.9828, -33.4123) (-12.9859, -33.4232) knots 0 0 0 0 0 0 0.022222 0.044444 0.066667 0.088889 0.111111 0.133333 0.155556 0.177778 0.2 0.222222 0.244444 0.266667 0.288889 0.311111 0.333333 0.355556 0.377778 0.4 0.422222 0.444444 0.466667 0.488889 0.511111 0.533333 0.555556 0.577778 0.6 0.622222 0.644444 0.666667 0.688889 0.711111 0.733333 0.755556 0.777778 0.8 0.822222 0.844444 0.866667 0.888889 0.911111 0.933333 0.955556 0.977778 1 1 1 1 1 1
  arc A60 (-12.9859, -33.4232) -> (-12.6425, -33.7593) centre (0, -20.5) ccw
  circle A61 centre (0, -20.5) radius 2.9
  circle A62 centre (0, -20.5) radius 6
  line L0 (-12.5, -55.5) -> (12.5, -55.5)
  line L1 (0, -55.5) -> (0, -20.5) construction
  line L2 (12.5, 14.5) -> (-12.5, 14.5)
  line L3 (-12.5, 14.5) -> (-12.5, -55.5)
  line L4 (-12.5, -55.5) -> (12.5, -55.5)
  line L5 (12.5, -55.5) -> (12.5, 14.5)
  line L6 (12.5, 14.5) -> (-12.5, -55.5) construction
  line L7 (-12.5, 14.5) -> (12.5, -55.5) construction
  point P0 (0, -20.5)
  dimension "d91" = 5.8
  dimension "d92" = 12
  dimension "d93" = 25
  dimension "d94" = 70
  constraint concentric A0 A61
  constraint concentric A61 A62
  constraint midpoint L0 L1.start
  constraint coincident P0 A0.centre
  constraint horizontal L2
  constraint perpendicular L2 L3
  constraint parallel L2 L4
  constraint parallel L3 L5
  constraint coincident L6 P0
  constraint coincident L7 P0
  measures "d91" diameter of A61
  measures "d92" diameter of A62
  measures "d93" distance of L0.start L0.end
  measures "d94" distance of L2.end L0.start
extrude "Extrude1" add sketch "Sketch1" along normal blind 7 contours A0 | A61 | A62
sketch "Sketch2" plane through (0, 0, -8.25) normal (0, 0, -1) x (1, 0, 0)
  circle A0 centre (0, 0) radius 6
  circle A1 centre (8.2191, -28.465) radius 1.725
  circle A2 centre (-7.8309, -12.415) radius 1.725
  circle A3 centre (8.1691, -12.415) radius 1.725
  circle A4 centre (-7.8309, -28.465) radius 1.725
  arc A5 (11.6441, -12.4041) -> (8.1691, -8.94) centre (8.1691, -12.415) ccw
  line L0 (8.1691, -8.94) -> (-7.8309, -8.94)
  arc A6 (-7.8309, -8.94) -> (-11.3059, -12.415) centre (-7.8309, -12.415) ccw
  line L1 (-11.3059, -12.415) -> (-11.3059, -28.465)
  arc A7 (-11.3059, -28.465) -> (-7.8309, -31.94) centre (-7.8309, -28.465) ccw
  line L2 (-7.8309, -31.94) -> (8.2191, -31.94)
  arc A8 (8.2191, -31.94) -> (11.6941, -28.4541) centre (8.2191, -28.465) ccw
  line L3 (11.6941, -28.4541) -> (11.6441, -12.4041)
  line L4 (-11.4059, -12.415) -> (-11.4059, -28.465)
  arc A9 (-11.4059, -28.465) -> (-7.8309, -32.04) centre (-7.8309, -28.465) ccw
  line L5 (-7.8309, -32.04) -> (8.2191, -32.04)
  arc A10 (8.2191, -32.04) -> (11.7941, -28.4538) centre (8.2191, -28.465) ccw
  line L6 (11.7941, -28.4538) -> (11.7441, -12.4038)
  arc A11 (11.7441, -12.4038) -> (8.1691, -8.84) centre (8.1691, -12.415) ccw
  line L7 (8.1691, -8.84) -> (-7.8309, -8.84)
  arc A12 (-7.8309, -8.84) -> (-11.4059, -12.415) centre (-7.8309, -12.415) ccw
  line L8 (-12.5, -35) -> (12.5, -35)
  line L9 (-12.5, -35) -> (-12.5, 6)
  line L10 (-12.5, 6) -> (12.5, 6)
  line L11 (12.5, 6) -> (12.5, -35)
  point P0 (-12.5, -35)
  dimension "d97" = 0.1
  dimension "d1" = 41
  dimension "d2" = 25
  dimension "d3" = 3.06
  dimension "d4" = 1.0941
  dimension "d5" = 0.8059
  dimension "d6" = 8.84
  dimension "d7" = 3.475
  constraint coincident P0 L8.start
  constraint perpendicular L8 L9
  constraint perpendicular L9 L10
  constraint coincident L8.end L11.end
  constraint perpendicular L10 L11
  constraint tangent A0 L10
  measures "d1" distance of L10.end L8.end
  measures "d2" distance of P0 L8.end
  measures "d3" distance of L2 L8
  measures "d4" distance of L4 L9
  measures "d5" distance of A8.end L11
  measures "d6" distance of A0.centre L7
  measures "d7" distance of A2.centre L0.end
extrude "Extrude2" add sketch "Sketch2" against normal blind 6 contours L8 L9 L10 L11
sketch "Sketch3" plane through (0, -6, 0) normal (0, -1, 0) x (1, 0, 0)
  line L0 (-12.5, -8.25) -> (12.5, -8.25)
  line L1 (12.5, -8.25) -> (12.5, -2.25)
  line L2 (12.5, -2.25) -> (0, -2.25)
  line L3 (0, -2.25) -> (-12.5, -2.25)
  line L4 (-12.5, -2.25) -> (-12.5, -8.25)
  circle A0 centre (25, 13.25) radius 3
  circle A1 centre (-25, 13.25) radius 3
  circle A2 centre (-25, 13.25) radius 5
  circle A3 centre (25, 13.25) radius 5
  line L5 (12.5, -2.25) -> (20, -2.25)
  line L6 (20, -2.25) -> (20, 13.25)
  line L7 (12.5, -8.25) -> (26, -8.25)
  line L8 (26, -8.25) -> (26, 13.25)
  line L9 (28.5355, 9.7145) -> (26, 7.1789)
  line L10 (0, -8.25) -> (0, -2.25)
  line L11 (-26, -8.25) -> (-26, 13.25)
  line L12 (-20, -2.25) -> (-20, 13.25)
  line L13 (-12.5, -2.25) -> (-20, -2.25)
  line L14 (-12.5, -8.25) -> (-26, -8.25)
  circle A4 centre (-25, 13.25) radius 5
  line L15 (-28.5355, 9.7145) -> (-26, 7.1789)
  point P0 (-12.5, -2.25)
  dimension "d100" = 2
  dimension "d101" = 2
  dimension "d103" = 6
  dimension "d104" = 45
  constraint coincident L1.end L2.start
  constraint perpendicular L1 L5
  constraint coincident A3 L6.end
  constraint tangent A3 L6
  constraint perpendicular L5 L6
  constraint coincident A3 L9.start
  constraint coincident L8 L9.end
  constraint tangent A3 L9
  constraint midpoint L0 L10.start
  constraint coincident L2.end L3.start
  constraint symmetric A3 L10 A4
  constraint symmetric L1.end L10 P0
  constraint symmetric L5.end L10 L12.start
  constraint symmetric L6.end L10 L12.end
  constraint symmetric L0.end L10 L0.start
  constraint symmetric L7.end L10 L11.start
  constraint symmetric L8.end L10 L11.end
  constraint symmetric L9.start L10 L15.start
  constraint symmetric L9.end L10 L15.end
  constraint coincident P0 L3.end
  constraint concentric A2 A4
  measures "d104" angle of L8 L9
extrude "Extrude3" add sketch "Sketch3" along normal blind 10 from surface at -21 contours L4 A2 L11 L12 L13 L14 A4 | L1 A3 L5 L6 L7 L8 | A2 L11 A4 L15 | A2 A4 | A3 L8 L9 | A3
extrude "Extrude4" cut 2 faces at (24, 15, -1.107) (-24, 15, -1.107) along direction (0, -1, 0) blind 0.1
extrude "Extrude5" add sketch "Sketch1" against normal blind 1.9 contours A61
